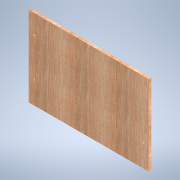
# Autodesk Inventor part: Seite_links
Saved by Autodesk Inventor 2021 (Build 250183000, 183)
## iProperties
Created: 2022-06-26
Part Number: Seite_links
Material: Holz (Birke)
Document SubType Name: Modeling
Designer: adria
Density: 0.55 g/cm^3
Appearance: Birke - natur - poliert
Mass: 3295.18 g
Surface Area: 7933.08 cm^2
Volume: 5991.24 cm^3
Author: adria
Autodesk Inventor part; units mm, degrees
ref_plane "YZ Plane" through (0, 0, 0) normal (1, 0, 0) x (0, 1, 0)
ref_plane "XZ Plane" through (0, 0, 0) normal (0, 1, 0) x (-1, 0, 0)
ref_plane "XY Plane" through (0, 0, 0) normal (0, 0, 1) x (1, 0, 0)
sketch "Skizze1" plane through (0, 0, 0) normal (0, 0, 1) x (1, 0, 0)
  line L0 (-375, -250) -> (375, -250)
  line L1 (375, -250) -> (375, 250)
  line L2 (375, 250) -> (-375, 250)
  line L3 (-375, 250) -> (-375, -250)
  line L4 (-375, -250) -> (375, 250) construction
  line L5 (375, -250) -> (-375, 250) construction
  point P0 (0, 0)
  dimension "d0" = 750
  dimension "d1" = 500
  constraints: 12 end point, 2 midpoint, 2 parallel, 1 horizontal, 1 perpendicular
  measures "d0" distance of L2.end L1.end
  measures "d1" distance of L1.end L0.end
extrude "Extrusion1" add sketch "Skizze1" along normal blind 16
sketch "Skizze5" plane through (0, 0, 16) normal (0, 0, 1) x (1, 0, 0)
  line L0 (375, -250) -> (375, 250) projected
  line L1 (375, 250) -> (-375, 250) projected
  line L2 (-375, 250) -> (-375, -250) projected
  line L3 (-375, -250) -> (375, -250) projected
  point P0 (0, 0)
  point P1 (340, -110)
  point P2 (-340, -110)
  point P3 (-340, 130)
  dimension "d39" = 140
  dimension "d40" = 140
  dimension "d41" = 35
  dimension "d42" = 35
  dimension "d44" = 120
  dimension "d57" = 35
  measures "d39" distance from line of L3 point (-340, -110)
  measures "d40" distance from line of L3 point (340, -110)
  measures "d41" distance from line of L0 point (340, -110)
  measures "d42" distance from line of L2 point (-340, -110)
  measures "d44" distance from line of L1 point (-340, 130)
  measures "d57" distance from line of L2 point (-340, 130)
hole "Bohrung4" at (340, -110, 16) at (-340, -110, 16) at (-340, 130, 16) direction (0, 0, -1) diameter 10 end through all
sketch "Skizze9" plane through (0, 0, 0) normal (0, 0, -1) x (-1, 0, 0)
  line L0 (-375, -250) -> (-375, 250) projected
  line L1 (375, -250) -> (-375, -250) projected
  point P0 (0, 0)
  point P1 (-150, -74.5)
  point P2 (-130, -54.5)
  point P3 (-130, -94.5)
  point P4 (-110, -74.5)
  dimension "d101" = 40
  dimension "d102" = 40
  dimension "d103" = 20
  dimension "d104" = 20
  dimension "d105" = 175.5
  dimension "d106" = 245
  constraints: 1 horizontal alignment, 1 vertical alignment
  measures "d101" distance of point (-130, -54.5) point (-130, -94.5)
  measures "d102" distance of point (-110, -74.5) point (-150, -74.5)
  measures "d103" horizontal distance of point (-110, -74.5) point (-130, -94.5)
  measures "d104" horizontal distance of point (-130, -94.5) point (-110, -74.5)
  measures "d105" distance from line of L1 point (-110, -74.5)
  measures "d106" distance from line of L0 point (-130, -94.5)
hole "Bohrung8" at (150, -74.5, 0) at (130, -54.5, 0) at (130, -94.5, 0) at (110, -74.5, 0) direction (0, 0, 1) diameter 4.4 end through all
sketch "Skizze10" plane through (0, 0, 0) normal (0, 0, -1) x (-1, 0, 0)
  line L0 (-375, -250) -> (-375, 250) projected
  line L1 (375, -250) -> (-375, -250) projected
  line L2 (375, 250) -> (375, -250) projected
  line L3 (-375, 250) -> (375, 250) projected
  point P0 (0, 0)
  point P1 (-367, 242)
  point P2 (0, 242)
  point P3 (367, 242)
  point P4 (-367, -242)
  point P5 (37, -242)
  dimension "d114" = 8
  dimension "d115" = 8
  dimension "d116" = 8
  dimension "d118" = 8
  dimension "d128" = 338
  constraints: 3 horizontal alignment, 2 vertical alignment
  measures "d114" distance from line of point (-367, 242) L3
  measures "d115" distance from line of L0 point (-367, 242)
  measures "d116" distance from line of L1 point (-367, -242)
  measures "d118" distance from line of L2 point (367, 242)
  measures "d128" distance from line of L2 point (37, -242)
hole "Bohrung9" at (367, 242, 0) at (0, 242, 0) at (-367, 242, 0) at (367, -242, 0) at (-37, -242, 0) direction (0, 0, 1) diameter 8 depth 20 tip angle 118
equation "\"d116\" = d114"
equation "\"d118\" = d115"
